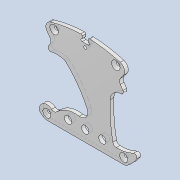
# Autodesk Inventor part: 脚中間フレーム外v2
Saved by Autodesk Inventor 2020 (Build 240168000, 168)
## iProperties
Created: 2021-02-23
Part Number: 脚中間フレーム外v2
Material: アルミニウム 2014-T4
Document SubType Name: Modeling
Designer: AA19065
Density: 2.8 g/cm^3
Appearance: サテン
Author: AA19065
Autodesk Inventor part; units mm, degrees
ref_plane "YZ Plane" through (0, 0, 0) normal (1, 0, 0) x (0, 1, 0)
ref_plane "XZ Plane" through (0, 0, 0) normal (0, 1, 0) x (-1, 0, 0)
ref_plane "XY Plane" through (0, 0, 0) normal (0, 0, 1) x (1, 0, 0)
sketch "スケッチ1" plane through (0, 0, 0) normal (0, 0, 1) x (1, 0, 0)
  circle A0 centre (82.5564, 47.1333) radius 1.5
  circle A1 centre (133, 47.1333) radius 1.5
  circle A2 centre (76.6032, -15) radius 1.25
  circle A3 centre (139.3968, -15) radius 1.25
  circle A4 centre (104.0735, 2) radius 6.025
  circle A5 centre (137.3222, 20) radius 9.0064
  circle A6 centre (133.5, -8) radius 3
  circle A7 centre (82.5, -8) radius 3
  circle A8 centre (90, 27) radius 3
  arc A9 (90.8877, 29.8657) -> (71.1185, 25.1885) centre (84.9697, 10.7613) ccw
  circle A10 centre (90, 27) radius 3
  arc A11 (109.5592, 4.4914) -> (92.0759, 29.1658) centre (36.7191, -28.5891) ccw
  circle A12 centre (104.0735, 2) radius 6.025
  circle A13 centre (82.5, -8) radius 3
  arc A14 (80.5672, -10.2944) -> (70.6533, -16.5669) centre (76.6032, -15) ccw
  arc A15 (128.3227, 20.3537) -> (130.5559, -8.5765) centre (253.2262, 15.4443) ccw
  circle A16 centre (137.3222, 20) radius 9.0064
  arc A17 (142.297, -19.0729) -> (142.6609, 27.2536) centre (125.7093, 4.222) ccw
  arc A18 (136.6782, 35.3358) -> (180.0662, 10.7187) centre (180.8617, 62.6652) ccw
  arc A19 (133.4146, -10.9988) -> (152.9487, -4.4855) centre (134.2687, 18.9891) ccw
  circle A20 centre (133.5, -8) radius 3
  arc A21 (79.4181, 50.9264) -> (76.8573, 42.9425) centre (80.8701, 46.058) ccw
  arc A22 (136.5819, 50.9264) -> (79.4181, 50.9264) centre (108, -44.902) ccw
  arc A23 (139.1427, 42.9425) -> (136.5819, 50.9264) centre (135.1299, 46.058) ccw
  line L0 (135.1299, 46.058) -> (140.08, 37.44) construction
  arc A24 (167.8386, 64.1653) -> (136.7771, 39.6963) centre (191.2716, 2.4693) ccw
  circle A25 centre (140.08, 37.44) radius 4
  arc A26 (136.8078, 35.1273) -> (180.0662, 10.7187) centre (180.8617, 62.6652) ccw
  circle A27 centre (75.92, 37.44) radius 4
  arc A28 (79.2229, 39.6963) -> (48.1614, 64.1653) centre (24.7284, 2.4693) ccw
  arc A29 (35.9338, 10.7187) -> (79.3218, 35.3358) centre (35.1383, 62.6652) ccw
  line L1 (105.5, 50.098) -> (105.5, 57.098)
  line L2 (110.5, 50.098) -> (105.5, 50.098)
  line L3 (110.5, 57.098) -> (110.5, 50.098)
  line L4 (76.6032, -20) -> (139.3968, -20)
  arc A30 (142.297, -19.0729) -> (142.6609, 27.2536) centre (125.7093, 4.222) ccw
  arc A31 (73.3391, 27.2536) -> (73.703, -19.0729) centre (90.2907, 4.222) ccw
  circle A32 centre (76.6032, -15) radius 5
  circle A33 centre (94, -11) radius 1.5
  circle A34 centre (108, -11) radius 1.5
  circle A35 centre (122, -11) radius 1.5
  circle A36 centre (139.3968, -15) radius 5
  arc A37 (91.1836, 30.8209) -> (70.426, 25.9099) centre (84.9697, 10.7613) ccw
  circle A38 centre (90, 27) radius 4
  arc A39 (110.4697, 4.9049) -> (92.7678, 29.8877) centre (36.7191, -28.5891) ccw
  circle A40 centre (104.0735, 2) radius 7.025
  circle A41 centre (82.5, -8) radius 4
  arc A42 (79.9229, -11.0592) -> (72.6057, -18.2512) centre (76.6032, -15) ccw
  circle A43 centre (137.3222, 20) radius 10.0064
  arc A44 (127.3234, 20.393) -> (129.5746, -8.7687) centre (253.2262, 15.4443) ccw
  circle A45 centre (133.5, -8) radius 4
  arc A46 (133.3861, -11.9984) -> (153.5714, -5.268) centre (134.2687, 18.9891) ccw
  arc A47 (149.962, -10.931) -> (148.0243, -8.7919) centre (148.6899, -10.1362) ccw
  circle A48 centre (94, -11) radius 3
  circle A49 centre (108, -11) radius 3
  circle A50 centre (122, -11) radius 3
  arc A51 (78.0489, 33.3777) -> (79.6666, 31.0807) centre (79.2878, 32.5321) ccw
  arc A52 (137.4162, 30.006) -> (138.6491, 32.3803) centre (137.4303, 31.5059) ccw
  arc A53 (103.1113, -3.9477) -> (84.6572, -10.0848) centre (99.758, -24.6782) ccw
  arc A54 (102.9517, -4.9349) -> (85.3763, -10.7797) centre (99.758, -24.6782) ccw
  line L5 (108, 72.8318) -> (108, -27.6373) construction
  line L6 (110.5, 57.098) -> (110.5, 50.098)
  line L7 (110.5, 50.098) -> (105.5, 50.098)
  line L8 (105.5, 50.098) -> (105.5, 57.098)
  arc A55 (105.5, 52.198) -> (105.5, 50.098) centre (105.5, 51.148) ccw
  line L9 (105.5, 50.098) -> (105.5, 51.148) construction
  line L10 (105.5, 52.198) -> (105.5, 51.148) construction
  arc A56 (110.5, 50.098) -> (110.5, 52.198) centre (110.5, 51.148) ccw
  line L11 (110.5, 50.098) -> (110.5, 51.148) construction
  line L12 (110.5, 52.198) -> (110.5, 51.148) construction
  line L13 (105.5, 57.098) -> (105.5, 44.098)
  line L14 (105.5, 44.098) -> (110.5, 44.098)
  line L15 (110.5, 44.098) -> (110.5, 57.098)
  circle A57 centre (108, 47.098) radius 1.25
  point P0 (0, 0)
  point P1 (86.8725, 16.8134)
  point P2 (144.2273, 7.0155)
  point P3 (129.1275, 16.8134)
  point P4 (147.2589, -13)
  point P5 (133.2785, 1.3235)
  point P6 (127.5476, 8.263)
  point P7 (132.4267, -7.6361)
  point P8 (94, -9)
  point P9 (108, -9)
  point P10 (122, -9)
  point P11 (96, 42)
  point P12 (120, 42)
  point P13 (138.7615, 30.8147)
  point P14 (105.5, 55.0668)
  point P15 (92.7678, 29.8877)
  point P16 (102.9517, -4.9349)
  point P17 (85.3763, -10.7797)
  point P18 (149.962, -10.931)
  point P19 (129.5746, -8.7687)
  point P20 (138.6491, 32.3803)
  point P21 (110.5, 55.0668)
  point P22 (143.3172, 26.7558)
  point P23 (108, -14.5)
  point P24 (108, 57.098)
  dimension "d0" = 1
  dimension "d1" = 1
  dimension "d2" = 1
  dimension "d3" = 1
  dimension "d4" = 1
  dimension "d5" = 1
  dimension "d6" = 1
  dimension "d7" = 1
  dimension "d8" = 1
  dimension "d9" = 1
  dimension "d10" = 1.5
  dimension "d11" = 6
  dimension "d12" = 6
  dimension "d13" = 6
  dimension "d14" = 1.5
  dimension "d15" = 1
  dimension "d24" = 5
  dimension "d25" = 1.05
  dimension "d26" = 180
  dimension "d27" = 1.05
  dimension "d28" = 180
  dimension "d29" = 13
  dimension "d30" = 2.5
  dimension "d31" = 3
  constraints: 68 point on circle, 54 centre point, 32 end point, 7 tangent, 5 point on line, 4 vertical, 3 coincident, 2 horizontal, 2 parallel, 1 equal radius, 47 other
  measures "d0" radial gap between concentric circles of A9 A37
  measures "d2" radial gap between concentric circles of A11 A39
  measures "d3" radial gap between concentric circles of A4 A40
  measures "d4" radial gap between concentric circles of A7 A41
  measures "d5" radial gap between concentric circles of A14 A42
  measures "d7" radial gap between concentric circles of A15 A44
  measures "d8" radial gap between concentric circles of A6 A45
  measures "d9" radial gap between concentric circles of A19 A46
  measures "d10" radius of A47
  measures "d11" diameter of A48
  measures "d12" diameter of A49
  measures "d13" diameter of A50
  measures "d14" radius of A51
  measures "d15" radial gap between concentric circles of A53 A54
  measures "d24" distance between parallel lines of L6 L8
  measures "d25" radius of A55
  measures "d26" angle of L9 L10
  measures "d27" radius of A56
  measures "d28" angle of L11 L12
  measures "d29" distance of L15.start L6.start
  measures "d30" diameter of A57
  measures "d31" distance from line of L14 A57.centre
extrude "押し出し1" add sketch "スケッチ1" along normal blind 3 contours A4 A11 A40 A53 | A11 A38 A39 A40 | A40 A54 A41 A53 | A11 A8 A9 A38 | A39 A38 A37 A51 A29 A27 A28 A21 A22 L1 A55 L13 L14 L15 A56 L3 A23 A24 A25 A18 A52 A43 A44 A45 A46 A36 L4 A32 A31 A42 A41 A54 A40 | A41 A14 A7 A53 | A9 A29 A37 A38 | A42 A31 A14 A41 | A37 A29 A51 | A32 | A36 A46 | A36 A46 A47 A17 | A46 A45 A19 A36 | A36 A19 A46 | A47 A46 A17 | A45 A15 A6 A19 | A36 A19 A17 A46 | A44 A43 A15 A45 | A43 A18 A17 A5 A15 | L2 L15 L14 L13 | A52 A18 A43 picked at (110.6939, 1.4268) picked at (92.7442, 29.3928) picked at (85.317, -10.3143) picked at (129.8786, -8.3803)
chamfer "面取り1" distance 2 angle 45 4 edges at (81.0564, 47.1333, 3) (131.5, 47.1333, 3) (75.3532, -15, 3) (138.1468, -15, 3)
fillet "フィレット1" radius 2 4 edges at (70.6533, -16.5669, 1.5) (152.9487, -4.4855, 1.5) (143.3172, 26.7558, 1.5) (71.1185, 25.1885, 1.5)
fillet "フィレット2" radius 1 2 edges at (105.5, 55.0668, 1.5) (110.5, 55.0668, 1.5)
